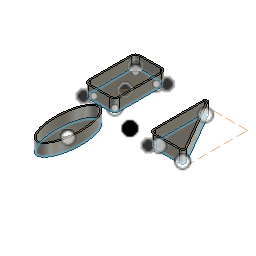
3Organs (Autodesk Fusion 360 design; units mm, degrees)
part number: 2026-05-30-11-02-58-227
part number: 2026-06-04-07-38-33-386
part number: 2026-06-04-07-38-33-413
part number: 2026-06-04-07-38-33-432
Autodesk Fusion 360 part; units mm, degrees
note: some values were not read from the file. Chosen so that the rebuilt part matches the saved one: which bodies a step acts on.
sketch "OrganRect" plane through (0, 0, 0) normal (0, 0, 1) x (1, 0, 0)
  line L0 (-44.1863, 54.6026) -> (-24.1863, 54.6026)
  line L1 (-19.1863, 49.6026) -> (-19.1863, 9.6026)
  line L2 (-24.1863, 4.6026) -> (-44.1863, 4.6026)
  line L3 (-49.1863, 9.6026) -> (-49.1863, 49.6026)
  arc A0 (-49.1863, 9.6026) -> (-44.1863, 4.6026) centre (-44.1863, 9.6026) ccw
  arc A1 (-24.1863, 4.6026) -> (-19.1863, 9.6026) centre (-24.1863, 9.6026) ccw
  arc A2 (-44.1863, 54.6026) -> (-49.1863, 49.6026) centre (-44.1863, 49.6026) ccw
  arc A3 (-19.1863, 49.6026) -> (-24.1863, 54.6026) centre (-24.1863, 49.6026) ccw
  line L4 (-34.1863, 54.6026) -> (-34.1863, 4.6026) construction
  line L5 (-49.1863, 29.6026) -> (-19.1863, 29.6026) construction
  arc A4 (-44.1863, 53.1026) -> (-47.6863, 49.6026) centre (-44.1863, 49.6026) ccw
  line L6 (-47.6863, 9.6026) -> (-47.6863, 49.6026)
  arc A5 (-47.6863, 9.6026) -> (-44.1863, 6.1026) centre (-44.1863, 9.6026) ccw
  line L7 (-24.1863, 6.1026) -> (-44.1863, 6.1026)
  arc A6 (-24.1863, 6.1026) -> (-20.6863, 9.6026) centre (-24.1863, 9.6026) ccw
  line L8 (-20.6863, 49.6026) -> (-20.6863, 9.6026)
  arc A7 (-20.6863, 49.6026) -> (-24.1863, 53.1026) centre (-24.1863, 49.6026) ccw
  line L9 (-44.1863, 53.1026) -> (-24.1863, 53.1026)
  point P0 (-49.1863, 54.6026)
  point P1 (-19.1863, 54.6026)
  point P2 (-49.1863, 4.6026)
  point P3 (-34.1863, 29.6026)
  dimension "d20" = 30
  dimension "d21" = 50
  dimension "d22" = 5
  dimension "d39" = 1.5
  constraint horizontal L0
  constraint vertical L1
  constraint horizontal L2
  constraint vertical L3
  constraint coincident P2 L2
  constraint coincident P2 L3
  constraint tangent L2 A0
  constraint tangent L3 A0
  constraint tangent L1 A1
  constraint tangent L2 A1
  constraint equal A0 A1
  constraint coincident P0 L0
  constraint coincident P0 L3
  constraint tangent L0 A2
  constraint tangent L3 A2
  constraint equal A0 A2
  constraint coincident P1 L0
  constraint coincident P1 L1
  constraint tangent L0 A3
  constraint tangent L1 A3
  constraint equal A0 A3
  constraint midpoint L0 L4.start
  constraint midpoint L2 L4.end
  constraint midpoint L3 L5.start
  constraint midpoint L1 L5.end
  constraint midpoint L5 P3
  measures "d20" distance of P0 P1
  measures "d21" distance of P0 P2
  measures "d22" radius of A0
sketch "OrganTriang" plane through (0, 0, 0) normal (0, 0, 1) x (1, 0, 0)
  line L0 (28.0195, -5.2298) -> (52.7964, -5.2298)
  line L1 (58.0195, -5.2298) -> (58.0195, 54.7702) construction
  line L2 (58.0195, 54.7702) -> (23.0195, 54.7702) construction
  line L3 (23.0195, 47.3724) -> (23.0195, -0.2298)
  line L4 (26.7471, 48.3801) -> (55.3877, -0.7182)
  arc A0 (26.7471, 48.3801) -> (23.0195, 47.3724) centre (25.0195, 47.3724) ccw
  arc A1 (23.0195, -0.2298) -> (28.0195, -5.2298) centre (28.0195, -0.2298) ccw
  arc A2 (52.7964, -5.2298) -> (55.3877, -0.7182) centre (52.7964, -2.2298) ccw
  line L5 (40.4079, -5.2298) -> (40.4079, 24.9615) construction
  line L6 (23.0195, 23.5713) -> (40.4079, 23.5713) construction
  line L7 (28.0195, -3.7298) -> (52.7964, -3.7298)
  arc A3 (52.7964, -3.7298) -> (54.0921, -1.474) centre (52.7964, -2.2298) ccw
  line L8 (25.4514, 47.6243) -> (54.0921, -1.474)
  arc A4 (25.4514, 47.6243) -> (24.5195, 47.3724) centre (25.0195, 47.3724) ccw
  line L9 (24.5195, 47.3724) -> (24.5195, -0.2298)
  arc A5 (24.5195, -0.2298) -> (28.0195, -3.7298) centre (28.0195, -0.2298) ccw
  point P0 (23.0195, -5.2298)
  dimension "d23" = 35
  dimension "d24" = 60
  dimension "d25" = 2
  dimension "d26" = 5
  dimension "d27" = 3
  constraint horizontal L0
  constraint vertical L1
  constraint horizontal L2
  constraint vertical L3
  constraint coincident L2.end L3
  constraint coincident L2.end L4
  constraint tangent L3 A0
  constraint tangent L4 A0
  constraint coincident P0 L0
  constraint coincident P0 L3
  constraint tangent L0 A1
  constraint tangent L3 A1
  constraint coincident L1.start L4
  constraint coincident L1.start L0
  constraint tangent L4 A2
  constraint tangent L0 A2
  constraint midpoint L0 L5.start
  constraint coincident L4 L5.end
  constraint perpendicular L0 L5
  constraint midpoint L3 L6.start
  constraint coincident L5 L6.end
  constraint perpendicular L5 L6
  measures "d23" distance of P0 L1.start
  measures "d24" distance of P0 L2.end
  measures "d25" radius of A0
  measures "d26" radius of A1
  measures "d27" radius of A2
sketch "OrganElipse" plane through (0, 0, 0) normal (0, 0, 1) x (1, 0, 0)
  ellipse E0 centre (-22.0664, -37.4011) end of major axis (-22.0664, -67.4011) minor radius 12.5
  line L0 (-22.0664, -7.4011) -> (-22.0664, -67.4011) construction
  line L1 (-34.5664, -37.4011) -> (-9.5664, -37.4011) construction
  ellipse E1 centre (-22.0664, -37.4011) end of major axis (-22.0664, -65.9011) minor radius 11
  dimension "d28" = 60
  dimension "d29" = 25
  constraint coincident E0 L0.start
  constraint coincident E0 L0.end
  constraint coincident E0 L1.start
  constraint coincident E0 L1.end
  constraint vertical L0
  measures "d28" distance of E0
extrude "Extrude3" add sketch "OrganRect" sketch "OrganElipse" sketch "OrganTriang" along normal blind 1.5 contours A4 L6 A5 L7 A6 L8 A7 L9 of sketch 2 contours E1 of sketch 3 contours L7 A3 L8 A4 L9 A5 makes body 1 at (-25.6628, -37.1882, 0) makes body 2 at (-29.6863, 22.936, 0) makes body 3 at (34.6876, 15.3069, 0)
extrude "Extrude5" add sketch "OrganRect" sketch "OrganTriang" sketch "OrganElipse" along normal blind 11.5 of sketch 2 of sketch 3 bodies 3 2 1
copy_body "Body->Comp10" bodies 3 removing the originals makes body 4 in component "OrganTriang"
copy_body "Body->Comp11" bodies 2 removing the originals makes body 5 in component "OrganRect"
copy_body "Body->Comp12" bodies 1 removing the originals makes body 6 in component "OrganElipse"
component "OrganTriang" placed x (1, 0, 0) y (0, 1, 0) z (0, 0, 1) at (0, 0, 0)
component "OrganRect" placed x (1, 0, 0) y (0, 1, 0) z (0, 0, 1) at (0, 0, 0)
component "OrganElipse" placed x (1, 0, 0) y (0, 1, 0) z (0, 0, 1) at (0, 0, 0)
equation "WallThickness = 1.5 mm"
equation "Tolerances = 0.5 mm"
equation "d34 = WallThickness"
equation "d39 = WallThickness"
equation "d40 = -WallThickness"
equation "d43 = 10 mm + WallThickness"
